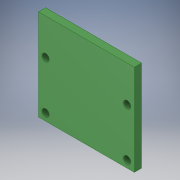
# Autodesk Inventor part: CameraBoard
Saved by Autodesk Inventor 2018 (Build 220112000, 112)
## iProperties
Created: 2018-01-13
Part Number: CameraBoard
Material: Thermoplastic Resin
Document SubType Name: Modeling
Designer: Kyle-HP
Density: 1.28 g/cm^3
Appearance: Smooth - Dark Forest Green
Author: Kyle-HP
Autodesk Inventor part; units mm, degrees
ref_plane "YZ Plane" through (0, 0, 0) normal (1, 0, 0) x (0, 1, 0)
ref_plane "XZ Plane" through (0, 0, 0) normal (0, 1, 0) x (-1, 0, 0)
ref_plane "XY Plane" through (0, 0, 0) normal (0, 0, 1) x (1, 0, 0)
sketch "Sketch1" plane through (0, 0, 0) normal (0, 0, 1) x (1, 0, 0)
  line L0 (0, 0) -> (25.4, 0)
  line L1 (25.4, 0) -> (25.4, -24.13)
  line L2 (25.4, -24.13) -> (0, -24.13)
  line L3 (0, -24.13) -> (0, 0)
  dimension "d0" = 25.4
  dimension "d1" = 24.13
  constraints: 8 end point, 2 parallel, 1 horizontal, 1 perpendicular
  measures "d0" distance of L0.start L0.end
  measures "d1" distance of L0.end L1.end
extrude "Extrusion1" add sketch "Sketch1" along normal blind 1.905
sketch "Sketch2" plane through (0, 0, 1.905) normal (0, 0, 1) x (1, 0, 0)
  circle A0 centre (1.905, -22.225) radius 0.9525
  circle A1 centre (1.905, -9.525) radius 0.9525
  circle A2 centre (23.495, -9.525) radius 0.9525
  circle A3 centre (23.495, -22.225) radius 0.9525
  line L0 (25.4, -24.13) -> (25.4, 0) projected
  line L1 (0, -24.13) -> (25.4, -24.13) projected
  line L2 (0, 0) -> (0, -24.13) projected
  line L3 (25.4, 0) -> (0, 0) projected
  dimension "d4" = 1.905
  dimension "d5" = 1.905
  dimension "d6" = 1.905
  dimension "d7" = 1.905
  dimension "d8" = 1.905
  dimension "d9" = 1.905
  dimension "d10" = 1.905
  dimension "d11" = 1.905
  dimension "d12" = 9.525
  dimension "d13" = 9.525
  dimension "d14" = 1.905
  dimension "d15" = 1.905
  constraints: 4 centre point
  measures "d4" diameter of A3
  measures "d5" diameter of A2
  measures "d6" diameter of A1
  measures "d7" diameter of A0
  measures "d8" distance from line of A3.centre L0
  measures "d9" distance from line of L1 A3.centre
  measures "d10" distance from line of L2 A0.centre
  measures "d11" distance from line of L1 A0.centre
  measures "d12" distance from line of L3 A2.centre
  measures "d13" distance from line of L3 A1.centre
  measures "d14" distance from line of L2 A1.centre
  measures "d15" distance from line of L0 A2.centre
extrude "Extrusion2" cut sketch "Sketch2" against normal blind 1.905 contours A0 | A1 | A2 | A3
body "Solid1"
